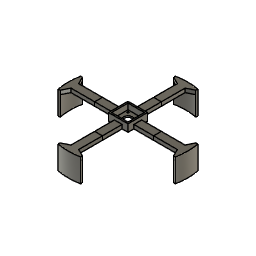
Stirrer Holder v3 (Autodesk Fusion 360 design; units mm, degrees)
Autodesk Fusion 360 part; units mm, degrees
sketch "Sketch1" plane through (0, 0, 0) normal (0, 0, 1) x (1, 0, 0)
  circle A0 centre (0, 0) radius 137.5
  circle A1 centre (0, 0) radius 149
  circle A2 centre (0, 0) radius 154
  line L0 (0, 0) -> (-10, 0)
  line L1 (-10, 0) -> (-10, -153.675)
  line L2 (0, 0) -> (10, 0)
  line L3 (10, 0) -> (10, -153.675)
  line L4 (0, 0) -> (29.3846, -151.1706)
  line L5 (0, 0) -> (154, 0) construction
  line L6 (0, 0) -> (-29.3846, -151.1706)
  line L7 (0, 0) -> (154, 0) construction
  line L8 (28.4305, -146.2625) -> (10, -137.1359)
  line L9 (-28.4305, -146.2625) -> (-10, -137.1359)
  line L10 (0, 0) -> (21.15, 0)
  line L11 (0, 0) -> (-21.15, 0)
  line L12 (21.15, 0) -> (-21.15, 0)
  line L13 (-21.15, 0) -> (-21.15, -21.15)
  line L14 (-21.15, -21.15) -> (21.15, -21.15)
  line L15 (21.15, -21.15) -> (21.15, 0)
  circle A3 centre (0, 0) radius 11.2
  line L16 (-21.15, -21.15) -> (-15.35, -21.15)
  line L17 (-15.35, -21.15) -> (-15.35, -15.35)
  line L18 (-15.35, -15.35) -> (-21.15, -15.35)
  line L19 (-21.15, -15.35) -> (-21.15, -21.15)
  line L20 (21.15, -21.15) -> (15.35, -21.15)
  line L21 (15.35, -21.15) -> (15.35, -15.35)
  line L22 (15.35, -15.35) -> (21.15, -15.35)
  line L23 (21.15, -15.35) -> (21.15, -21.15)
  circle A4 centre (15.35, -15.35) radius 2
  circle A5 centre (-15.35, -15.35) radius 2
  line L24 (25.15, -25.15) -> (25.15, 4)
  line L25 (25.15, 4) -> (-25.15, 4)
  line L26 (-25.15, 4) -> (-25.15, -25.15)
  line L27 (-25.15, -25.15) -> (25.15, -25.15)
  point P0 (0, 149)
  dimension "d1" = 275
  dimension "d2" = 298
  dimension "d3" = 308
  dimension "d4" = 10
  dimension "d5" = 79
  dimension "d7" = 101
  dimension "d21" = 21.15
  dimension "d22" = 21.15
  dimension "d23" = 21.15
  dimension "d24" = 22.4
  dimension "d25" = 5.8
  dimension "d26" = 5.8
  dimension "d27" = 5.8
  dimension "d28" = 5.8
  dimension "d29" = 4
  dimension "d30" = 4
  dimension "d31" = 4
  constraint coincident A0.centre A1.centre
  constraint concentric A0 A1
  constraint concentric A0 A2
  constraint horizontal L0
  constraint coincident A2 L1.end
  constraint perpendicular L0 L1
  constraint perpendicular L1 L2
  constraint coincident A2 L3.end
  constraint perpendicular L2 L3
  constraint horizontal L5
  constraint horizontal L7
  constraint coincident A2 L6.end
  constraint coincident A2 L4.end
  constraint coincident L4 L8.start
  constraint coincident A1 L8.start
  constraint coincident A0 L8.end
  constraint coincident L3 L8.end
  constraint coincident L6 L9.start
  constraint coincident A1 L9.start
  constraint coincident A0 L9.end
  constraint coincident L1 L9.end
  constraint equal L0 L2
  constraint perpendicular L3 L10
  constraint parallel L0 L11
  constraint horizontal L12
  constraint vertical L13
  constraint horizontal L14
  constraint vertical L15
  constraint horizontal L16
  constraint vertical L17
  constraint horizontal L18
  constraint vertical L19
  constraint horizontal L20
  constraint vertical L21
  constraint horizontal L22
  constraint vertical L23
  constraint coincident L21.end L22.start
  constraint coincident L17.end L18.start
  measures "d1" diameter of A0
  measures "d2" diameter of A1
  measures "d3" diameter of A2
  measures "d4" distance of A0.centre L2.end
  measures "d5" angle of L4 L5
  measures "d7" angle of L6 L7
  measures "d21" distance of A0.centre L10.end
  measures "d22" distance of A0.centre L11.end
  measures "d23" distance of L10.end L14.end
  measures "d24" diameter of A3
  measures "d25" distance of L13.end L18.end
  measures "d26" distance of L13.end L16.end
  measures "d27" distance of L14.end L20.end
  measures "d28" distance of L14.end L22.end
  measures "d29" diameter of A4
  measures "d30" diameter of A5
extrude "Extrude1" add sketch "Sketch1" along normal blind 10 contours A0 L1 L3 L4 L6 L27 | A0 A1 L1 L3 | A1 L1 L9 | A1 L3 L8 | L1 L6 L27 | A1 A2 L1 L6 | A1 A2 L1 L3 | L3 L4 L27 | A1 A2 L3 L4 | L1 L11 L12 L13 L14 A3 L16 L19 L25 L26 L27 | L1 L6 L14 L27 | L4 L6 L14 L27 | L3 L4 L14 L27 | L3 L10 L12 L14 L15 A3 L20 L23 L24 L25 L27 | L1 L11 L12 L13 L14 A3 L17 L18 A5 | L1 L6 L14 A3 | L4 L6 L14 A3 | L3 L4 L14 A3 | L3 L10 L12 L14 L15 A3 L21 L22 A4 | L13 L14 L16 L17 L18 L19 A5 | L14 L15 L20 L21 L22 L23 A4 makes body 1
extrude "Extrude2" add sketch "Sketch1" against normal blind 50 contours A1 A2 L1 L6 | A1 A2 L1 L3 | A1 A2 L3 L4 bodies 1
ref_plane "WorkPlane1" through (-17.8057, -76, 5) normal (0, 1, 0) x (-1, 0, 0)
split "Split1" by plane through (-17.8057, -76, 5) normal (0, 1, 0) bodies 1 makes body 2 at (3.3333, -59.05, 10)
sketch "Sketch2" plane through (0, -76, 0) normal (0, -1, 0) x (1, 0, 0)
  line L0 (-10, 0) -> (10, 0)
  line L1 (10, 0) -> (10, 10)
  line L2 (10, 10) -> (-10, 10)
  line L3 (-10, 10) -> (-10, 0)
  line L4 (-7, 3) -> (7, 3)
  line L5 (7, 3) -> (7, 7)
  line L6 (7, 7) -> (-7, 7)
  line L7 (-7, 7) -> (-7, 3)
  line L8 (-6.6, 3.4) -> (6.6, 3.4)
  line L9 (6.6, 3.4) -> (6.6, 6.6)
  line L10 (6.6, 6.6) -> (-6.6, 6.6)
  line L11 (-6.6, 6.6) -> (-6.6, 3.4)
  dimension "d15" = -3
  dimension "d16" = -3.4
extrude "Extrude3" add sketch "Sketch2" along normal blind 20 contours L8 L9 L10 L11 bodies 2
extrude "Extrude4" cut sketch "Sketch2" along normal blind 20.4 contours L4 L5 L6 L7 | L8 L9 L10 L11 bodies 1
pattern_circular "C-Pattern1" count 4 over 360 about axis through (0, 0, 1.75) along (0, 0, 1) of bodies 1 2 makes body 3 at (59.05, 3.3333, 10) makes body 4 at (-3.3333, 59.05, 10) makes body 5 at (-42.1, 3.3333, 10) makes body 6 at (153.1249, -16.3944, -10) makes body 7 at (16.3944, 153.1249, -10) makes body 8 at (-152.2863, -22.9103, -10)
combine "Combine2" operation add target body 3 tool bodies 4 5 2
copy_body "Body->Comp1" bodies 8 removing the originals makes body 9 in component "Outside"
copy_body "CutPasteBodies1" bodies 1 6 7 removing the originals makes body 10 makes body 11 makes body 12 in component "Outside"
copy_body "Body->Comp2" bodies 3 removing the originals makes body 13 in component "Center"
sketch "Sketch5" plane through (0, 0, 10) normal (0, 0, 1) x (-1, 0, 0)
  line L0 (-25.15, 10) -> (-76, 10)
  line L1 (-76, 10) -> (-76, -10)
  line L2 (-76, -10) -> (-25.15, -10)
  line L3 (-25.15, -10) -> (-25.15, -25.15)
  line L4 (-25.15, -25.15) -> (-10, -25.15)
  line L5 (-10, -25.15) -> (-10, -76)
  line L6 (-10, -76) -> (10, -76)
  line L7 (10, -76) -> (10, -25.15)
  line L8 (10, -25.15) -> (25.15, -25.15)
  line L9 (25.15, -25.15) -> (25.15, -10)
  line L10 (25.15, -10) -> (76, -10)
  line L11 (76, -10) -> (76, 10)
  line L12 (76, 10) -> (25.15, 10)
  line L13 (25.15, 10) -> (25.15, 25.15)
  line L14 (25.15, 25.15) -> (10, 25.15)
  line L15 (10, 25.15) -> (10, 76)
  line L16 (10, 76) -> (-10, 76)
  line L17 (-10, 76) -> (-10, 25.15)
  line L18 (-10, 25.15) -> (-25.15, 25.15)
  line L19 (-25.15, 25.15) -> (-25.15, 10)
  circle A0 centre (0, 0) radius 11.2
  line L20 (25.15, -25.15) -> (-25.15, -25.15)
  line L21 (-25.15, -25.15) -> (-25.15, 25.15)
  line L22 (-25.15, 25.15) -> (25.15, 25.15)
  line L23 (25.15, 25.15) -> (25.15, -25.15)
  circle A1 centre (15.35, 15.35) radius 2
  circle A2 centre (-15.35, 15.35) radius 2
  circle A3 centre (15.35, -15.35) radius 2
  circle A4 centre (-15.35, -15.35) radius 2
  constraint horizontal L20
  constraint vertical L21
  constraint horizontal L22
  constraint vertical L23
  constraint coincident L18.end L19.start
  constraint coincident L8.end L9.start
extrude "Extrude1'" cut sketch "Sketch5" against normal blind 6 contours L3 L4 L8 L9 L13 L14 L18 L19 L20 L21 L22 L23 | A1 | A2 | A3 | A4 bodies 13 in component "Center"
sketch "Sketch6" plane through (0, 0, 4) normal (0, 0, 1) x (-1, 0, 0)
  circle A0 centre (0, 0) radius 11.2
  line L0 (-10, 25.15) -> (-25.15, 25.15)
  line L1 (-25.15, 25.15) -> (-25.15, 10)
  line L2 (-25.15, 10) -> (-25.15, -10)
  line L3 (-25.15, -10) -> (-25.15, -25.15)
  line L4 (-25.15, -25.15) -> (-10, -25.15)
  line L5 (-10, -25.15) -> (10, -25.15)
  line L6 (10, -25.15) -> (25.15, -25.15)
  line L7 (25.15, -25.15) -> (25.15, -10)
  line L8 (25.15, -10) -> (25.15, 10)
  line L9 (25.15, 10) -> (25.15, 25.15)
  line L10 (25.15, 25.15) -> (10, 25.15)
  line L11 (10, 25.15) -> (-10, 25.15)
  line L12 (21.15, -21.15) -> (21.15, -10)
  line L13 (21.15, -10) -> (21.15, 10)
  line L14 (21.15, 10) -> (21.15, 21.15)
  line L15 (21.15, 21.15) -> (10, 21.15)
  line L16 (10, 21.15) -> (-10, 21.15)
  line L17 (-10, 21.15) -> (-21.15, 21.15)
  line L18 (-21.15, 21.15) -> (-21.15, 10)
  line L19 (-21.15, 10) -> (-21.15, -10)
  line L20 (-21.15, -10) -> (-21.15, -21.15)
  line L21 (-21.15, -21.15) -> (-10, -21.15)
  line L22 (-10, -21.15) -> (10, -21.15)
  line L23 (10, -21.15) -> (21.15, -21.15)
  circle A1 centre (15.35, 15.35) radius 2
  circle A2 centre (15.35, -15.35) radius 2
  circle A3 centre (-15.35, -15.35) radius 2
  circle A4 centre (-15.35, 15.35) radius 2
  dimension "d34" = -4
extrude "Extrude2'" add sketch "Sketch6" along normal blind 15 contours L0 L1 L2 L3 L4 L5 L6 L7 L8 L9 L10 L11 bodies 13 in component "Center"
component "Outside" placed x (1, 0, 0) y (0, 1, 0) z (0, 0, 1) at (0, 0, 0)
component "Center" placed x (1, 0, 0) y (0, 1, 0) z (0, 0, 1) at (0, 0, 0)
equation "d3 = 298 mm + 10 mm"
equation "d21 = ( ( 41.9 + 0.4 ) / 2 ) * 1 mm"
equation "d22 = ( ( 41.9 + 0.4 ) / 2 ) * 1 mm"
equation "d23 = ( ( 41.9 + 0.4 ) / 2 ) * 1 mm"
named bodies: "Outside 4", "Center", "Outside 3", "Outside 2", "Outside"
